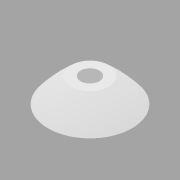
# Autodesk Inventor part: Cap
Saved by Autodesk Inventor 2019 (Build 230136000, 136)
## iProperties
Created: 2020-01-30
Part Number: Cap
Material: Generic
Document SubType Name: Modeling
Designer: alb16148
Density: 1 g/cm^3
Appearance: Default
Author: alb16148
## iProperties of the stored document Cap_3DPrint.ipt
Part Number: Cap_3DPrint
Material: Generic
Document SubType Name: Modeling
Designer: gfb14170
Appearance: Default
Author: gfb14170
Autodesk Inventor part; units mm, degrees
ref_plane "YZ Plane" through (0, 0, 0) normal (1, 0, 0) x (0, 1, 0)
ref_plane "XZ Plane" through (0, 0, 0) normal (0, 1, 0) x (-1, 0, 0)
ref_plane "XY Plane" through (0, 0, 0) normal (0, 0, 1) x (1, 0, 0)
sketch "Sketch1" plane through (0, 0, 0) normal (1, 0, 0) x (0, 1, 0)
  line L0 (121, 3) -> (1, 3)
  line L1 (1, 3) -> (1, -3)
  line L2 (1, -3) -> (121, -3)
  line L3 (121, -3) -> (121, 3)
  line L4 (121, 3) -> (1, -3) construction
  line L5 (1, 3) -> (121, -3) construction
  line L6 (10, 8.35) -> (0, 8.35)
  line L7 (0, 8.35) -> (0, 20)
  line L8 (10, 8.35) -> (10, 9.45)
  line L9 (10, 9.45) -> (16, 9.45)
  line L10 (16, 9.45) -> (16, 17)
  line L11 (16, 17) -> (18, 17)
  line L12 (18, 17) -> (18, 18.5)
  line L13 (18, 18.5) -> (16, 18.5)
  line L14 (16, 18.5) -> (16, 20)
  line L15 (16, 20) -> (0, 20)
  line L16 (-24.2, 0) -> (145.2, 0) projected
  line L17 (16, 20) -> (31, 20)
  line L18 (18, 17) -> (31, 17)
  line L19 (75, 9.45) -> (69, 9.45)
  line L20 (69, 9.45) -> (69, 8.35)
  line L21 (69, 8.35) -> (66, 8.35)
  line L22 (75, 9.45) -> (75, 12.45)
  arc A0 (75, 12.45) -> (31, 20) centre (31, -111.9869) ccw
  arc A1 (59.1084, 13.9001) -> (31, 17) centre (31, -111.9869) ccw
  arc A2 (66, 8.35) -> (59.1084, 13.9001) centre (56.9292, 4.1404) ccw
  line L23 (76, 13.45) -> (76, 7.5)
  line L24 (76, 7.5) -> (80, 7.5)
  line L25 (81, 6.5) -> (81, 3)
  arc A3 (81, 6.5) -> (80, 7.5) centre (80, 6.5) ccw
  line L26 (83.8376, 3) -> (83.8376, 6)
  arc A4 (83.8376, 6) -> (76, 13.45) centre (42.4933, -29.6477) ccw
  point P0 (0, 0)
  point P1 (61, 0)
  point P2 (61, 0)
  point P3 (81, 7.5)
  dimension "d0" = 120
  dimension "d1" = 6
  dimension "d5" = 8.35
  dimension "d6" = 9.45
  dimension "d7" = 1.5
  dimension "d8" = 1.5
  dimension "d9" = 20
  dimension "d10" = 6
  dimension "d11" = 2
  dimension "d13" = 10
  dimension "d14" = 1
  dimension "d15" = 6
  dimension "d16" = 3
  dimension "d17" = 9.45
  dimension "d18" = 3
  dimension "d19" = 8.35
  dimension "d20" = 15
  dimension "d21" = 7.55
  dimension "d22" = 75
  dimension "d23" = 10
  dimension "d25" = 5
  dimension "d26" = 1
  dimension "d27" = 7.5
  dimension "d28" = 1
  dimension "d32" = 6
  dimension "d33" = 1.5
  dimension "d34" = 1
  constraints: 52 end point, 10 point on circle, 9 perpendicular, 8 horizontal, 5 centre point, 5 tangent, 5 vertical, 4 point on line, 3 midpoint, 2 parallel, 2 vertical alignment, 1 collinear, 1 concentric, 1 horizontal alignment
  measures "d0" distance of L2.end L1.end
  measures "d1" distance of L1.end L0.end
  measures "d5" distance between parallel lines of L16 L6
  measures "d6" distance between parallel lines of L16 L9
  measures "d7" distance between parallel lines of L15 L13
  measures "d8" distance between parallel lines of L13 L11
  measures "d9" distance between parallel lines of L16 L15
  measures "d10" distance of L8.end L9.end
  measures "d11" distance of L12.end L13.end
  measures "d13" distance of L6.start L6.end
  measures "d14" distance from line of point (0, 0) L1
  measures "d15" distance of L19.start L19.end
  measures "d16" distance of L19.start L22.end
  measures "d17" distance between parallel lines of L16 L19
  measures "d18" distance of L20.end L21.end
  measures "d19" distance between parallel lines of L16 L21
  measures "d20" distance of L14.end L17.end
  measures "d21" distance of L9.end L10.end
  measures "d22" distance between parallel lines of L7 L22
  measures "d23" radius of A2
  measures "d25" distance of L23.end point (81, 7.5)
  measures "d26" distance between parallel lines of L22 L23
  measures "d27" distance between parallel lines of L24 L16
  measures "d28" radius of A3
  measures "d32" distance from line of L16 L26.end
  measures "d34" horizontal distance of L23.start L22.end
revolve "Revolution2" add sketch "Sketch1" angle 360 about axis through (0, -10, 0) along (0, 1, 0) contours L0 L25 A3 L24 L23 A4 L26
body "Solid2"
